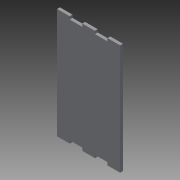
# Autodesk Inventor part: tapa supp
Saved by Autodesk Inventor 2015 (Build 190159000, 159)
## iProperties
Created: 2016-01-26
Part Number: tapa supp
Material: Generic
Document SubType Name: Modeling
Designer: iberopuebla
Density: 1 g/cm^3
Appearance: Default
Author: iberopuebla
Autodesk Inventor part; units mm, degrees
ref_plane "YZ Plane" through (0, 0, 0) normal (1, 0, 0) x (0, 1, 0)
ref_plane "XZ Plane" through (0, 0, 0) normal (0, 1, 0) x (-1, 0, 0)
ref_plane "XY Plane" through (0, 0, 0) normal (0, 0, 1) x (1, 0, 0)
sketch "Sketch1" plane through (0, 0, 0) normal (0, 1, 0) x (-1, 0, 0)
  line L0 (400, 0) -> (400, -700)
  line L1 (0, -700) -> (0, 0)
  line L2 (320, -682) -> (320, -700)
  line L3 (240, -682) -> (240, -700)
  line L4 (160, -682) -> (160, -700)
  line L5 (320, 0) -> (320, -18)
  line L6 (240, 0) -> (240, -18)
  line L7 (160, 0) -> (160, -18)
  line L8 (80, 0) -> (80, -18)
  line L9 (80, -682) -> (80, -700)
  line L10 (320, -682) -> (240, -682)
  line L11 (160, -682) -> (80, -682)
  line L12 (80, -700) -> (0, -700)
  line L13 (400, -700) -> (320, -700)
  line L14 (240, -700) -> (160, -700)
  line L15 (320, -18) -> (240, -18)
  line L16 (160, -18) -> (80, -18)
  line L17 (0, 0) -> (80, 0)
  line L18 (160, 0) -> (240, 0)
  line L19 (320, 0) -> (400, 0)
  dimension "d60" = 700
  dimension "d61" = 400
  dimension "d64" = 80
  dimension "d65" = 80
  dimension "d66" = 80
  dimension "d67" = 80
  dimension "d69" = 80
  dimension "d70" = 80
  dimension "d71" = 80
  dimension "d72" = 18
  constraints: 40 end point, 27 perpendicular, 10 parallel, 8 horizontal
  measures "d60" distance of L0.start L0.end
  measures "d61" distance of L1.end L0.start
  measures "d64" distance between parallel lines of L0 L2
  measures "d65" distance between parallel lines of L3 L2
  measures "d66" distance between parallel lines of L4 L3
  measures "d67" distance between parallel lines of L5 L0
  measures "d69" distance between parallel lines of L7 L6
  measures "d70" distance between parallel lines of L8 L7
  measures "d71" distance between parallel lines of L9 L4
  measures "d72" distance from line of L0.end L10
extrude "Extrusion1" add sketch "Sketch1" along normal blind 18
body "Solid1"
